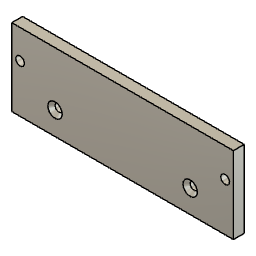
vector and synthrotek rail bracket (Autodesk Fusion 360 design; units mm, degrees)
Autodesk Fusion 360 part; units mm, degrees
note: some values were not read from the file. Set by a fixed rule: the direction of a hole.
sketch "Sketch2" plane through (0, 0, 0) normal (0, 0, 1) x (1, 0, 0)
  line L0 (-65.0875, 12.7) -> (65.0875, 12.7)
  line L1 (65.0875, 12.7) -> (65.0875, -12.7)
  line L2 (65.0875, -12.7) -> (-65.0875, -12.7)
  line L3 (-65.0875, -12.7) -> (-65.0875, 12.7)
  line L4 (-65.0875, 0) -> (65.0875, 0) construction
  line L5 (0, 12.7) -> (0, -12.7) construction
  line L6 (-65.0875, -12.7) -> (65.0875, -12.7)
  line L7 (65.0875, -12.7) -> (65.0875, -32.512)
  line L8 (65.0875, -32.512) -> (-65.0875, -32.512)
  line L9 (-65.0875, -32.512) -> (-65.0875, -12.7)
  point P0 (-60.2107, 0)
  point P1 (60.2107, 0)
  point P2 (-39.6875, -19.05)
  point P3 (-60.2107, -4.3713)
  point P4 (60.2107, -4.3713)
  point P5 (39.6875, -19.05)
  dimension "d2" = 25.4
  dimension "d3" = 120.4214
  dimension "d4" = 130.175
  dimension "d18" = 25.4
  dimension "d20" = 4.3713
  dimension "d23" = 19.05
  dimension "d24" = 19.812
  constraint horizontal L0
  constraint vertical L1
  constraint horizontal L2
  constraint vertical L3
  constraint horizontal P0 P1
  constraint midpoint L3 L4.start
  constraint midpoint L1 L4.end
  constraint coincident P1 L4
  constraint midpoint L0 L5.start
  constraint midpoint L2 L5.end
  constraint symmetric P0 P1 L5
  constraint midpoint L4 origin
  constraint vertical P0 P3
  constraint symmetric L5 P3 P4
  constraint horizontal L6
  constraint vertical L7
  constraint horizontal L8
  constraint vertical L9
  constraint coincident L2.end L3.start
  constraint collinear L1 L7
  constraint symmetric L5 P2 P5
  measures "d2" distance of L0.start L2.end
  measures "d3" distance of P0 P1
  measures "d4" distance of L0.start L0.end
  measures "d18" distance of L3 P2
  measures "d20" distance of P0 P3
  measures "d23" distance of L4 P2
  measures "d24" distance of L2 L8
extrude "Extrude1" add sketch "Sketch2" along normal blind 6.35
hole "Hole1" at (-60.2107, -4.3713, 0) at (60.2107, -4.3713, 0) direction (0, 0, 1) diameter 5.1054 end through all
hole "Hole2" at (-39.6875, -19.05, 0) at (39.6875, -19.05, 0) direction (0, 0, 1) diameter 4.4958 depth 7.62 tip angle 118 countersink diameter 8.4328 countersink angle 82
move_body "Move1" bodies 1 to x (-1, 0, 0) y (0, 1, 0) z (0, 0, -1) at (0, 0, 0)
equation "synthrotek_spacing = 4.741 in"
equation "tiptop_spacing = 4.823 in"
